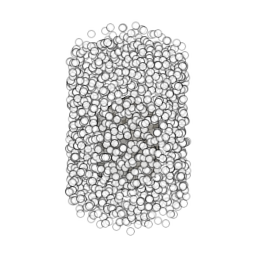
HALS-Total (Autodesk Fusion 360 archive; units mm, degrees)
design "PointCloud-1443points"
Autodesk Fusion 360 part; units mm, degrees
ref_plane "WorkPlane1" through (0, 0, 1223) normal (0, 0, 1) x (1, 0, 0)
sketch "CSV Points - Sketch1" plane through (0, 0, 0) normal (0, 0, 1) x (1, 0, 0)
  point P0 (142.14, 15.69)
  point P1 (141.12, 15.83)
  point P2 (134.47, 12)
  point P3 (116.13, 14.26)
  point P4 (129.36, 12.91)
  point P5 (124.41, 25.54)
  point P6 (141.97, 34.08)
  point P7 (106.73, 16.52)
  point P8 (125.57, 18.99)
  point P9 (134.24, 31.98)
  point P10 (130.24, 26.97)
  point P11 (146.5, 27.15)
  point P12 (98.71, 25.71)
  point P13 (125.11, 21.83)
  point P14 (125.91, 16.58)
  point P15 (113.34, 24.71)
  point P16 (145.3, 33.01)
  point P17 (131.67, 18.74)
  point P18 (136.19, 22.3)
  point P19 (135.78, 34.11)
  point P20 (143.32, 27.86)
  point P21 (129.53, 25.41)
  point P22 (116.49, 28.83)
  point P23 (141.16, 22.86)
  point P24 (141.54, 20.4)
  point P25 (133.86, 50.31)
  point P26 (128.21, 38.95)
  point P27 (129.84, 36.98)
  point P28 (125.52, 49.7)
  point P29 (133.48, 45.44)
  point P30 (125.98, 42.64)
  point P31 (125.43, 49.92)
  point P32 (137.66, 38.7)
  point P33 (116.67, 35.67)
  point P34 (138.63, 51.83)
  point P35 (122.24, 44.25)
  point P36 (141.15, 44.5)
  point P37 (117.73, 31.99)
  point P38 (104.55, 42.88)
  point P39 (131.17, 42.87)
  point P40 (133.94, 47.17)
  point P41 (123.23, 47.3)
  point P42 (141.02, 41.5)
  point P43 (118.06, 34.52)
  point P44 (109.08, 42.31)
  point P45 (128.64, 62.46)
  point P46 (124.24, 55.32)
  point P47 (109.64, 60.03)
  point P48 (123.56, 67.93)
  point P49 (136.01, 60.84)
  point P50 (113.44, 54.84)
  point P51 (132.76, 67.64)
  point P52 (106.86, 45.14)
  point P53 (124.95, 65.32)
  point P54 (117.03, 67.3)
  point P55 (123.06, 57.91)
  point P56 (129.92, 59.75)
  point P57 (121.97, 68.73)
  point P58 (122.62, 65.47)
  point P59 (118.39, 51.23)
  point P60 (117.24, 58.45)
  point P61 (115.65, 57.16)
  point P62 (132.97, 57.82)
  point P63 (99.49, 53.57)
  point P64 (97.67, 54.81)
  point P65 (114.35, 85.86)
  point P66 (120.7, 87.37)
  point P67 (110.26, 74.37)
  point P68 (94.95, 57.5)
  point P69 (101.04, 60.95)
  point P70 (101.85, 68.96)
  point P71 (103.82, 74.87)
  point P72 (119.64, 90.48)
  point P73 (110.83, 71.7)
  point P74 (101.43, 64.12)
  point P75 (111.81, 79.17)
  point P76 (118.39, 81.98)
  point P77 (125.8, 74.1)
  point P78 (94.34, 58.49)
  point P79 (104.36, 68.81)
  point P80 (97.27, 71.97)
  point P81 (86.12, 63.5)
  point P82 (109.11, 72.49)
  point P83 (126.06, 77.55)
  point P84 (96.39, 93.08)
  point P85 (98.57, 86.29)
  point P86 (97.21, 84.8)
  point P87 (81.73, 79.48)
  point P88 (110.02, 86.58)
  point P89 (95.82, 78.71)
  point P90 (96.7, 89.86)
  point P91 (96.15, 87.49)
  point P92 (87.33, 73.28)
  point P93 (98.24, 75.66)
  point P94 (91.69, 90.74)
  point P95 (111.02, 94.82)
  point P96 (93.93, 83.98)
  point P97 (100.83, 95.68)
  point P98 (108.18, 87.29)
  point P99 (107.7, 86.28)
  point P100 (85.45, 81.38)
  point P101 (97.81, 87.15)
  point P102 (103.86, 89.34)
  point P103 (82.82, 96.28)
  point P104 (99.12, 111.25)
  point P105 (102.06, 107.18)
  point P106 (75.65, 94.43)
  point P107 (72.22, 89.5)
  point P108 (82.6, 87.04)
  point P109 (94.65, 105.86)
  point P110 (71.44, 83.64)
  point P111 (95.66, 96.67)
  point P112 (76.88, 99.83)
  point P113 (93.85, 111.84)
  point P114 (86.15, 94.67)
  point P115 (80.33, 86.44)
  point P116 (85.05, 103.55)
  point P117 (82.87, 105.3)
  point P118 (78.78, 81.01)
  point P119 (86.12, 98.72)
  point P120 (80.36, 91.79)
  point P121 (101.42, 105.02)
  point P122 (60.26, 97.95)
  point P123 (80.8, 121.61)
  point P124 (81.89, 111.08)
  point P125 (85.06, 114.95)
  point P126 (64.96, 98.51)
  point P127 (71.67, 115.59)
  point P128 (61.41, 104.26)
  point P129 (66.04, 95.37)
  point P130 (79.74, 112.63)
  point P131 (78.55, 124.25)
  point P132 (73.87, 114.19)
  point P133 (82.64, 109.27)
  point P134 (81.89, 113.55)
  point P135 (78.49, 115.93)
  point P136 (58.88, 97.61)
  point P137 (73.04, 120.61)
  point P138 (77.17, 114.41)
  point P139 (76.81, 106.12)
  point P140 (83.46, 111.16)
  point P141 (72.43, 129.07)
  point P142 (66.85, 124.15)
  point P143 (53.03, 121.97)
  point P144 (46.97, 95.03)
  point P145 (53.99, 108.29)
  point P146 (56.79, 131.24)
  point P147 (66.41, 124.38)
  point P148 (60.87, 108.03)
  point P149 (52.23, 113.56)
  point P150 (60.46, 128.49)
  point P151 (72.28, 125.7)
  point P152 (50.04, 95.71)
  point P153 (57.2, 135.41)
  point P154 (66.74, 130.98)
  point P155 (64.85, 134.15)
  point P156 (51.86, 115.93)
  point P157 (59.26, 107.79)
  point P158 (66.27, 121.05)
  point P159 (60.6, 136.12)
  point P160 (65.08, 134.03)
  point P161 (53.88, 138.92)
  point P162 (37.33, 127.65)
  point P163 (40.09, 136.22)
  point P164 (41.57, 108.3)
  point P165 (45.84, 130.16)
  point P166 (46.6, 142.58)
  point P167 (48.57, 118.43)
  point P168 (30.94, 113.87)
  point P169 (34.88, 110.63)
  point P170 (39.48, 109.07)
  point P171 (52.18, 139.56)
  point P172 (30.41, 99.46)
  point P173 (36.53, 129.96)
  point P174 (51.39, 129.15)
  point P175 (38.15, 112.72)
  point P176 (41.25, 121.17)
  point P177 (41.97, 105.99)
  point P178 (37.26, 130.8)
  point P179 (41.57, 136.82)
  point P180 (41.52, 110.46)
  point P181 (15.4, 106.9)
  point P182 (21.58, 133.26)
  point P183 (34.83, 140.75)
  point P184 (26.95, 137.38)
  point P185 (21.94, 112.89)
  point P186 (30.94, 123.17)
  point P187 (23.43, 143.09)
  point P188 (18.88, 132.66)
  point P189 (28.8, 126.77)
  point P190 (28.12, 128.97)
  point P191 (18.4, 105.41)
  point P192 (33.02, 126.77)
  point P193 (26.97, 145.52)
  point P194 (26.57, 128.28)
  point P195 (32.44, 136.19)
  point P196 (22.28, 147.32)
  point P197 (22.18, 143.29)
  point P198 (32.45, 135.16)
  point P199 (26.94, 131.26)
  point P200 (8.64, 126.71)
  point P201 (2.61, 135.97)
  point P202 (2.18, 124.98)
  point P203 (9.98, 142.65)
  point P204 (12.32, 123.39)
  point P205 (15.11, 123.08)
  point P206 (6.94, 141.83)
  point P207 (4.68, 121.91)
  point P208 (16.97, 128.89)
  point P209 (11.91, 133.47)
  point P210 (9.78, 121.61)
  point P211 (0.98, 140)
  point P212 (3.65, 122.95)
  point P213 (7.94, 137.77)
  point P214 (15.61, 139.13)
  point P215 (15.47, 140.15)
  point P216 (8.36, 136.74)
  point P217 (3.74, 142.95)
  point P218 (-6.64, 118.81)
  point P219 (-10.91, 148.6)
  point P220 (-12.75, 119.32)
  point P221 (-2.6, 123.97)
  point P222 (-3.64, 148.96)
  point P223 (-12.75, 121.33)
  point P224 (-9.82, 130.63)
  point P225 (-7.57, 139.8)
  point P226 (-16.26, 126.96)
  point P227 (-0.24, 136)
  point P228 (-5.76, 131.87)
  point P229 (-12.3, 143.47)
  point P230 (-12.8, 135.4)
  point P231 (-4.31, 129.93)
  point P232 (-1.44, 117.99)
  point P233 (-16.33, 139.04)
  point P234 (-8.67, 137.73)
  point P235 (-8.91, 137.71)
  point P236 (-15.63, 135.1)
  point P237 (-18.03, 120.66)
  point P238 (-22.14, 110.81)
  point P239 (-26.88, 133.32)
  point P240 (-20.89, 141.47)
  point P241 (-35.81, 140.51)
  point P242 (-33.32, 143.17)
  point P243 (-24.52, 144.94)
  point P244 (-24.08, 133.85)
  point P245 (-27.49, 123.99)
  point P246 (-33.68, 126.6)
  point P247 (-18.19, 132.76)
  point P248 (-30.36, 142.81)
  point P249 (-25.06, 132.65)
  point P250 (-22.93, 143.18)
  point P251 (-32.21, 133.16)
  point P252 (-34.11, 138.87)
  point P253 (-21.04, 134.36)
  point P254 (-28.18, 146.31)
  point P255 (-24.34, 116.49)
  point P256 (-32.54, 116.54)
  point P257 (-39.14, 131.29)
  point P258 (-47.6, 142.25)
  point P259 (-53.76, 137.89)
  point P260 (-50.21, 127.47)
  point P261 (-43.24, 130)
  point P262 (-40.81, 136.01)
  point P263 (-38.22, 137.8)
  point P264 (-41.13, 114.86)
  point P265 (-40.75, 110.74)
  point P266 (-42.82, 137.49)
  point P267 (-41.27, 128.54)
  point P268 (-45.7, 113.12)
  point P269 (-46.52, 122.46)
  point P270 (-46.46, 134.18)
  point P271 (-37.49, 130.73)
  point P272 (-41.6, 144.12)
  point P273 (-48.18, 139.94)
  point P274 (-49.94, 130.79)
  point P275 (-51.49, 102.83)
  point P276 (-61.55, 113.37)
  point P277 (-55.47, 126.36)
  point P278 (-56.09, 127.18)
  point P279 (-70.87, 131.07)
  point P280 (-62.9, 125.07)
  point P281 (-64.15, 134.49)
  point P282 (-60.94, 106.84)
  point P283 (-55.34, 132.94)
  point P284 (-57.26, 123.36)
  point P285 (-58.25, 112.85)
  point P286 (-59.9, 113.12)
  point P287 (-48.33, 106.55)
  point P288 (-58.07, 136.13)
  point P289 (-64.68, 116.21)
  point P290 (-58.74, 120.44)
  point P291 (-60.04, 122.03)
  point P292 (-68.36, 123.32)
  point P293 (-53.79, 124.91)
  point P294 (-56.98, 126.78)
  point P295 (-70.28, 112.91)
  point P296 (-79.36, 110.44)
  point P297 (-86.45, 116.41)
  point P298 (-64.71, 108.12)
  point P299 (-74.35, 111.48)
  point P300 (-72.51, 107.9)
  point P301 (-67.59, 113.38)
  point P302 (-87.46, 116.91)
  point P303 (-80.14, 112.35)
  point P304 (-60.41, 96.68)
  point P305 (-77.04, 120.47)
  point P306 (-84.89, 121.23)
  point P307 (-88.47, 116.14)
  point P308 (-70.42, 121)
  point P309 (-78.53, 114.69)
  point P310 (-79.94, 122.17)
  point P311 (-66.88, 109.14)
  point P312 (-82.49, 113.12)
  point P313 (-88, 120.24)
  point P314 (-71.9, 117.79)
  point P315 (-81.19, 93.73)
  point P316 (-90.62, 111.91)
  point P317 (-80.29, 83.72)
  point P318 (-88.76, 92.23)
  point P319 (-81.99, 100.89)
  point P320 (-80.37, 93.11)
  point P321 (-87.16, 96.46)
  point P322 (-78.63, 101)
  point P323 (-80.55, 87.6)
  point P324 (-95.08, 112.11)
  point P325 (-93.9, 113.1)
  point P326 (-98.65, 100.74)
  point P327 (-71.88, 76.54)
  point P328 (-93.17, 117.55)
  point P329 (-84.82, 95.87)
  point P330 (-89.94, 102.02)
  point P331 (-77.36, 96.91)
  point P332 (-94.64, 100.43)
  point P333 (-98.48, 100.91)
  point P334 (-110.9, 99.51)
  point P335 (-113.21, 98.41)
  point P336 (-87.82, 71.11)
  point P337 (-107, 102.25)
  point P338 (-94.39, 90.84)
  point P339 (-107.72, 87.85)
  point P340 (-111.28, 96.05)
  point P341 (-99.42, 89.84)
  point P342 (-108.1, 84.16)
  point P343 (-106, 97.47)
  point P344 (-91.92, 91.92)
  point P345 (-99.91, 84.73)
  point P346 (-112.33, 93.26)
  point P347 (-103.6, 101.45)
  point P348 (-102.06, 95.84)
  point P349 (-86.09, 68.48)
  point P350 (-106.35, 94.09)
  point P351 (-108.77, 95.89)
  point P352 (-96.13, 76.74)
  point P353 (-113.26, 67.79)
  point P354 (-108.15, 72.13)
  point P355 (-102.21, 68.42)
  point P356 (-115.96, 69.13)
  point P357 (-117.71, 88.06)
  point P358 (-105.02, 74.91)
  point P359 (-126.36, 78.96)
  point P360 (-112.05, 71.66)
  point P361 (-116.32, 81.45)
  point P362 (-90.68, 69.08)
  point P363 (-108.9, 63.38)
  point P364 (-104.79, 71.75)
  point P365 (-117.15, 76.66)
  point P366 (-110.84, 67.92)
  point P367 (-117.16, 85.43)
  point P368 (-120.24, 88)
  point P369 (-115.35, 70.14)
  point P370 (-114.51, 75.22)
  point P371 (-118.96, 81.15)
  point P372 (-116.34, 55.74)
  point P373 (-122.5, 61.34)
  point P374 (-116.77, 63.67)
  point P375 (-97.98, 43.01)
  point P376 (-132.67, 58.51)
  point P377 (-103.8, 56.12)
  point P378 (-104.43, 52.75)
  point P379 (-116.43, 55.54)
  point P380 (-107.71, 61.44)
  point P381 (-129.25, 53.8)
  point P382 (-121.54, 56.42)
  point P383 (-110.19, 56.87)
  point P384 (-98.1, 51.94)
  point P385 (-126.59, 57.42)
  point P386 (-125.1, 53.36)
  point P387 (-122.33, 68.09)
  point P388 (-129.32, 63.35)
  point P389 (-121.13, 59.6)
  point P390 (-120.7, 66.9)
  point P391 (-137.04, 40.85)
  point P392 (-109.06, 36.49)
  point P393 (-122.05, 47.59)
  point P394 (-129.42, 50.72)
  point P395 (-119.56, 39.77)
  point P396 (-142.72, 42.82)
  point P397 (-129.13, 35.81)
  point P398 (-116.82, 41.6)
  point P399 (-122.94, 45.23)
  point P400 (-125.07, 38.96)
  point P401 (-132.35, 42.49)
  point P402 (-113.12, 45.7)
  point P403 (-126.2, 47.94)
  point P404 (-137.96, 47.77)
  point P405 (-139.38, 39.97)
  point P406 (-131.56, 38.22)
  point P407 (-112.58, 38.55)
  point P408 (-136.39, 52.08)
  point P409 (-123.4, 49.61)
  point P410 (-142.14, 33.34)
  point P411 (-143.48, 36.31)
  point P412 (-146.37, 21.88)
  point P413 (-132.38, 26.45)
  point P414 (-116.65, 23.52)
  point P415 (-143.44, 21.18)
  point P416 (-137.54, 35.31)
  point P417 (-121.75, 28.33)
  point P418 (-120.29, 20.35)
  point P419 (-124.99, 22.49)
  point P420 (-136.68, 30.3)
  point P421 (-107.27, 28.54)
  point P422 (-147.62, 20.22)
  point P423 (-134.01, 28.48)
  point P424 (-129.7, 24.51)
  point P425 (-103.71, 16.43)
  point P426 (-113.67, 27.71)
  point P427 (-131.1, 32.2)
  point P428 (-118.56, 18.57)
  point P429 (-125.69, 24.2)
  point P430 (-130.26, 13.92)
  point P431 (-118.97, 2.7)
  point P432 (-146.96, 3.59)
  point P433 (-128.29, 13.48)
  point P434 (-144.59, 10.87)
  point P435 (-126.81, 6.87)
  point P436 (-116.08, 14.66)
  point P437 (-115, 0.2)
  point P438 (-122.88, 5.37)
  point P439 (-135.5, 11.62)
  point P440 (-142.37, 13.46)
  point P441 (-146.91, 5.13)
  point P442 (-138.99, 1.7)
  point P443 (-143.02, 16.8)
  point P444 (-107.79, 6.78)
  point P445 (-136.7, 9.08)
  point P446 (-115.25, 13.13)
  point P447 (-115.99, 1.62)
  point P448 (-112.94, 3.55)
  point P449 (-121.42, 11.91)
  point P450 (-138.02, -16.46)
  point P451 (-122.35, -12.64)
  point P452 (-138.68, -9.45)
  point P453 (-147.97, -2.84)
  point P454 (-144.98, -2.53)
  point P455 (-133.67, -9.35)
  point P456 (-145.28, -14.5)
  point P457 (-148.88, -18.28)
  point P458 (-125.85, -6.16)
  point P459 (-123.91, -4.76)
  point P460 (-145.4, -13.23)
  point P461 (-137.56, -11.07)
  point P462 (-132, -0.92)
  point P463 (-114.95, -3.41)
  point P464 (-115.8, -6.88)
  point P465 (-141.12, -15.83)
  point P466 (-141.14, -15.58)
  point P467 (-143.73, -8.79)
  point P468 (-146.95, -3.85)
  point P469 (-144.64, -35.79)
  point P470 (-124.62, -24.45)
  point P471 (-125.65, -24.42)
  point P472 (-128.99, -32.4)
  point P473 (-123.36, -20.2)
  point P474 (-119.79, -17.05)
  point P475 (-119.94, -27.25)
  point P476 (-117.25, -25.56)
  point P477 (-144.75, -19.06)
  point P478 (-110.33, -19.26)
  point P479 (-131.61, -34.28)
  point P480 (-140.65, -25.81)
  point P481 (-128.28, -26.57)
  point P482 (-137.16, -32.68)
  point P483 (-122.61, -18.54)
  point P484 (-132.42, -20.5)
  point P485 (-118.63, -28.48)
  point P486 (-130.28, -26.74)
  point P487 (-117.95, -22.07)
  point P488 (-138.62, -45.84)
  point P489 (-137.88, -48.01)
  point P490 (-106.28, -41.23)
  point P491 (-120.94, -35.36)
  point P492 (-110.32, -32.47)
  point P493 (-126.03, -48.38)
  point P494 (-133.94, -47.17)
  point P495 (-127.37, -41.63)
  point P496 (-98.07, -40.22)
  point P497 (-127.38, -34.61)
  point P498 (-140.12, -44.45)
  point P499 (-138.22, -50.04)
  point P500 (-113.34, -42.38)
  point P501 (-138.66, -42.39)
  point P502 (-134.71, -38.12)
  point P503 (-123.57, -49.18)
  point P504 (-128.82, -43.6)
  point P505 (-140.1, -47.7)
  point P506 (-105.99, -41.97)
  point P507 (-131.76, -37.53)
  point P508 (-98.13, -42.67)
  point P509 (-119.23, -58.93)
  point P510 (-127.98, -63.81)
  point P511 (-132.16, -57.19)
  point P512 (-96.06, -51.51)
  point P513 (-126.33, -71.18)
  point P514 (-119.01, -54.74)
  point P515 (-124.87, -58.76)
  point P516 (-118.75, -62.08)
  point P517 (-129.98, -54.64)
  point P518 (-117.61, -59.93)
  point P519 (-105.34, -50.92)
  point P520 (-106.8, -47.77)
  point P521 (-106.91, -58.77)
  point P522 (-129.82, -71.07)
  point P523 (-135.2, -60.2)
  point P524 (-125.04, -60.72)
  point P525 (-132.88, -67.41)
  point P526 (-127.26, -75.56)
  point P527 (-125.2, -77.03)
  point P528 (-101.62, -67.51)
  point P529 (-114.29, -84.27)
  point P530 (-119.77, -88.63)
  point P531 (-110.2, -72.66)
  point P532 (-124.08, -76.94)
  point P533 (-114.6, -67.5)
  point P534 (-103.59, -71.73)
  point P535 (-104.59, -73.78)
  point P536 (-103.06, -59.5)
  point P537 (-114.11, -72.14)
  point P538 (-123.42, -79.85)
  point P539 (-115, -86.66)
  point P540 (-97.33, -70.19)
  point P541 (-97.71, -66.16)
  point P542 (-127.58, -76.96)
  point P543 (-100.08, -60.61)
  point P544 (-112.75, -76.05)
  point P545 (-102.88, -74.47)
  point P546 (-103.56, -98.62)
  point P547 (-85.07, -68.15)
  point P548 (-113.62, -91.68)
  point P549 (-96.47, -91.55)
  point P550 (-80.51, -71.99)
  point P551 (-93.39, -80.05)
  point P552 (-97.38, -96.37)
  point P553 (-105.37, -81.15)
  point P554 (-86.56, -72.63)
  point P555 (-101.91, -93.05)
  point P556 (-106.22, -98.7)
  point P557 (-102, -83.78)
  point P558 (-116.31, -91.52)
  point P559 (-88.9, -86.45)
  point P560 (-109.27, -95.32)
  point P561 (-86.53, -75.75)
  point P562 (-81.29, -78.5)
  point P563 (-115.36, -91.11)
  point P564 (-106.02, -86.77)
  point P565 (-86.14, -105.24)
  point P566 (-89.25, -113.01)
  point P567 (-88.92, -92.08)
  point P568 (-94.85, -108.35)
  point P569 (-88.09, -100.98)
  point P570 (-103.18, -106.1)
  point P571 (-89.05, -113.16)
  point P572 (-88.86, -108.18)
  point P573 (-89.86, -96.7)
  point P574 (-70.8, -77.54)
  point P575 (-90.63, -108.01)
  point P576 (-75.05, -97.45)
  point P577 (-92.14, -93.11)
  point P578 (-78.74, -91.87)
  point P579 (-94.65, -105.86)
  point P580 (-80.54, -84.87)
  point P581 (-81.01, -100.39)
  point P582 (-80.03, -99.9)
  point P583 (-99.31, -104.28)
  point P584 (-84.44, -116.65)
  point P585 (-78.85, -116.89)
  point P586 (-74.6, -123.17)
  point P587 (-77.48, -128.44)
  point P588 (-61.11, -90.26)
  point P589 (-80.14, -111.12)
  point P590 (-68.01, -90.25)
  point P591 (-78.22, -120.91)
  point P592 (-73.21, -115.8)
  point P593 (-77.82, -110.31)
  point P594 (-71.16, -102.77)
  point P595 (-65.98, -112.01)
  point P596 (-72.19, -116.44)
  point P597 (-74.31, -112.7)
  point P598 (-75.54, -102.09)
  point P599 (-67.06, -90.95)
  point P600 (-69.17, -104.12)
  point P601 (-78.07, -126.91)
  point P602 (-76.07, -128.12)
  point P603 (-50.22, -98.99)
  point P604 (-57.22, -117.84)
  point P605 (-56.13, -126.07)
  point P606 (-64.83, -118.41)
  point P607 (-71.78, -130.57)
  point P608 (-49.41, -110.45)
  point P609 (-62.24, -128.75)
  point P610 (-56.29, -110.48)
  point P611 (-53.48, -127.22)
  point P612 (-61.16, -116.98)
  point P613 (-73, -126.44)
  point P614 (-62.16, -132.1)
  point P615 (-61.01, -132.64)
  point P616 (-70.2, -124.58)
  point P617 (-54.82, -102.23)
  point P618 (-58.38, -134.91)
  point P619 (-64.25, -128.87)
  point P620 (-55.83, -112.96)
  point P621 (-55.82, -128.39)
  point P622 (-40.82, -143.3)
  point P623 (-48.96, -123.66)
  point P624 (-45.44, -133.48)
  point P625 (-34.95, -103.25)
  point P626 (-47.7, -119.86)
  point P627 (-31.04, -109.69)
  point P628 (-40.93, -133.88)
  point P629 (-39.92, -106.78)
  point P630 (-50.04, -138.22)
  point P631 (-43.54, -137.26)
  point P632 (-38.54, -141.86)
  point P633 (-50.47, -123.05)
  point P634 (-40.39, -123.57)
  point P635 (-48.83, -138.65)
  point P636 (-52.32, -136.3)
  point P637 (-41.22, -140.06)
  point P638 (-41.26, -141.09)
  point P639 (-48.1, -124)
  point P640 (-47.03, -135.05)
  point P641 (-45.84, -138.62)
  point P642 (-25.57, -136.63)
  point P643 (-28.96, -141.06)
  point P644 (-29.41, -122.52)
  point P645 (-20.35, -131.43)
  point P646 (-21.68, -143.37)
  point P647 (-29.2, -122.57)
  point P648 (-28.8, -139.05)
  point P649 (-24.55, -133.77)
  point P650 (-32.52, -124.83)
  point P651 (-24.59, -140.87)
  point P652 (-29.82, -136.79)
  point P653 (-27.03, -118.97)
  point P654 (-18.04, -126.72)
  point P655 (-22.3, -136.19)
  point P656 (-28.99, -115.41)
  point P657 (-24.42, -125.65)
  point P658 (-27.34, -139.34)
  point P659 (-35.55, -143.67)
  point P660 (-3.66, -139.95)
  point P661 (-9.04, -147.72)
  point P662 (-14.7, -133.19)
  point P663 (-16.5, -147.08)
  point P664 (-8.66, -145.74)
  point P665 (-3.59, -120.95)
  point P666 (-0.95, -136)
  point P667 (-11.87, -147.52)
  point P668 (-12.05, -132.45)
  point P669 (-15.79, -119.96)
  point P670 (-5.26, -136.9)
  point P671 (-6.64, -135.84)
  point P672 (-15.84, -129.03)
  point P673 (-13.21, -132.34)
  point P674 (-9.63, -137.66)
  point P675 (-2.53, -144.98)
  point P676 (-2.73, -141.97)
  point P677 (-8.43, -123.71)
  point P678 (-14.6, -141.25)
  point P679 (-16.58, -139.02)
  point P680 (14.15, -144.31)
  point P681 (3.96, -125.94)
  point P682 (1.98, -141.99)
  point P683 (14.6, -128.17)
  point P684 (8.95, -134.7)
  point P685 (9.04, -143.72)
  point P686 (13.77, -117.19)
  point P687 (1.69, -137.99)
  point P688 (4.54, -129.92)
  point P689 (13.55, -143.36)
  point P690 (12.04, -140.48)
  point P691 (6.5, -148.86)
  point P692 (0.22, -127)
  point P693 (15.29, -121.04)
  point P694 (6.98, -128.81)
  point P695 (11.25, -149.58)
  point P696 (14.32, -136.25)
  point P697 (3.25, -132.96)
  point P698 (2.84, -124.97)
  point P699 (14.98, -140.2)
  point P700 (27.42, -142.38)
  point P701 (22.43, -143.25)
  point P702 (27.43, -111.68)
  point P703 (28.18, -115.61)
  point P704 (23.15, -146.18)
  point P705 (26.74, -141.5)
  point P706 (28.9, -135.96)
  point P707 (18.32, -133.75)
  point P708 (26.23, -98.57)
  point P709 (30.3, -136.68)
  point P710 (25.85, -143.69)
  point P711 (21.18, -125.22)
  point P712 (33.09, -142.2)
  point P713 (32.83, -127.85)
  point P714 (20.89, -141.47)
  point P715 (20.16, -99.99)
  point P716 (28.8, -144.15)
  point P717 (21.14, -141.43)
  point P718 (34.59, -136.69)
  point P719 (32.65, -139.22)
  point P720 (39.16, -97.42)
  point P721 (48.52, -127.05)
  point P722 (46, -134.34)
  point P723 (41.29, -142.12)
  point P724 (36.38, -126.89)
  point P725 (42.54, -122.84)
  point P726 (45.45, -119.66)
  point P727 (49.07, -121.46)
  point P728 (38.21, -119.02)
  point P729 (39.55, -126.98)
  point P730 (44.54, -121.07)
  point P731 (40.59, -113.99)
  point P732 (37.95, -136.84)
  point P733 (38.79, -129.31)
  point P734 (39.77, -119.56)
  point P735 (43.06, -109.86)
  point P736 (50.49, -129.51)
  point P737 (42.2, -126.13)
  point P738 (36.28, -121.71)
  point P739 (56.72, -102.33)
  point P740 (64.46, -131)
  point P741 (64.23, -131.11)
  point P742 (65.66, -117.96)
  point P743 (52.57, -123.26)
  point P744 (59.49, -131.14)
  point P745 (52.41, -98.98)
  point P746 (67.88, -131.52)
  point P747 (62.73, -135.15)
  point P748 (57.26, -137.56)
  point P749 (72.83, -127.69)
  point P750 (64.15, -134.49)
  point P751 (51.4, -101.75)
  point P752 (68.01, -125.79)
  point P753 (50.85, -115.28)
  point P754 (55.87, -127.28)
  point P755 (69.41, -127.31)
  point P756 (61.34, -122.5)
  point P757 (63.95, -133.47)
  point P758 (67.06, -98.31)
  point P759 (80.16, -122.03)
  point P760 (67.54, -111.08)
  point P761 (84.46, -115.4)
  point P762 (77.77, -106.65)
  point P763 (69.49, -113.4)
  point P764 (82.13, -125.51)
  point P765 (63.28, -92.41)
  point P766 (62.37, -107.17)
  point P767 (89.08, -116.93)
  point P768 (73.99, -105.67)
  point P769 (75.97, -118.79)
  point P770 (79.49, -127.21)
  point P771 (71.43, -100.14)
  point P772 (75.48, -100.89)
  point P773 (72.2, -121.11)
  point P774 (65.64, -98.06)
  point P775 (78.79, -118.14)
  point P776 (69.33, -115.84)
  point P777 (87.97, -110.19)
  point P778 (87.95, -99.76)
  point P779 (96.74, -109.35)
  point P780 (90.26, -113.48)
  point P781 (85.57, -91.12)
  point P782 (87.46, -89.31)
  point P783 (91.98, -110.79)
  point P784 (92.49, -109.06)
  point P785 (92.73, -100.85)
  point P786 (78.01, -100.21)
  point P787 (93.19, -103.13)
  point P788 (95.4, -110.52)
  point P789 (91.64, -112.37)
  point P790 (89.45, -92.95)
  point P791 (100.18, -104.83)
  point P792 (94.4, -116.57)
  point P793 (66.92, -76.98)
  point P794 (98.17, -109.41)
  point P795 (103.78, -101.27)
  point P796 (96.79, -91.21)
  point P797 (91.44, -72.99)
  point P798 (94.51, -83.33)
  point P799 (109.35, -96.74)
  point P800 (108.15, -85.72)
  point P801 (102.78, -96.52)
  point P802 (75.02, -73.46)
  point P803 (106.18, -88.15)
  point P804 (99.15, -84.08)
  point P805 (98.99, -98.99)
  point P806 (97.9, -90.02)
  point P807 (112.05, -87.23)
  point P808 (109.07, -98.55)
  point P809 (77.21, -66.65)
  point P810 (97.01, -78.83)
  point P811 (76.38, -73.5)
  point P812 (77.95, -74.75)
  point P813 (108.8, -88.1)
  point P814 (99.02, -85.77)
  point P815 (97.3, -59.4)
  point P816 (109.75, -80.32)
  point P817 (102.61, -74.83)
  point P818 (109.14, -66.88)
  point P819 (103.76, -67.9)
  point P820 (103.14, -70.62)
  point P821 (108.03, -62.88)
  point P822 (106.59, -81.2)
  point P823 (120.42, -84.32)
  point P824 (115.42, -73.81)
  point P825 (123.82, -77.37)
  point P826 (121.3, -86.52)
  point P827 (95.29, -71.28)
  point P828 (116.82, -69.64)
  point P829 (94.62, -63.58)
  point P830 (118.97, -79.34)
  point P831 (119.27, -71.38)
  point P832 (112.39, -83.47)
  point P833 (120.19, -86.36)
  point P834 (120.55, -75.04)
  point P835 (135.91, -61.08)
  point P836 (119.4, -51.42)
  point P837 (108.45, -60.12)
  point P838 (115.75, -56.95)
  point P839 (113.25, -55.23)
  point P840 (120.58, -67.11)
  point P841 (124.18, -52.97)
  point P842 (119.3, -54.12)
  point P843 (121.08, -64.11)
  point P844 (116.41, -60.08)
  point P845 (118.82, -55.16)
  point P846 (129.25, -53.8)
  point P847 (127.69, -72.83)
  point P848 (110.12, -52.52)
  point P849 (116.14, -58.41)
  point P850 (111.72, -60.4)
  point P851 (134.5, -59.32)
  point P852 (106.22, -46.63)
  point P853 (114.25, -62.03)
  point P854 (94.78, -47.46)
  point P855 (131.72, -50.3)
  point P856 (128.59, -44.28)
  point P857 (143.16, -41.32)
  point P858 (131.69, -37.76)
  point P859 (108.67, -37.63)
  point P860 (100.03, -38)
  point P861 (117.75, -47.58)
  point P862 (114.26, -36.68)
  point P863 (117.44, -36.58)
  point P864 (102.3, -37.64)
  point P865 (133.69, -47.87)
  point P866 (104.07, -28.86)
  point P867 (136.01, -40.81)
  point P868 (141.38, -47.03)
  point P869 (110.72, -43.61)
  point P870 (132.3, -51.58)
  point P871 (110.01, -36.81)
  point P872 (143.75, -42.85)
  point P873 (134.84, -37.65)
  point P874 (136.06, -28.42)
  point P875 (137.47, -26.47)
  point P876 (131.4, -20.58)
  point P877 (145.67, -35.78)
  point P878 (131.21, -31.74)
  point P879 (130.34, -20.88)
  point P880 (128.72, -24.32)
  point P881 (131.07, -27.86)
  point P882 (128.8, -17.64)
  point P883 (120.8, -32.14)
  point P884 (143.52, -31.82)
  point P885 (116.14, -20.9)
  point P886 (137.05, -23.18)
  point P887 (135.38, -31.5)
  point P888 (139.54, -35.57)
  point P889 (148.39, -21.91)
  point P890 (131.36, -26.49)
  point P891 (139.25, -27.82)
  point P892 (145.39, -21.73)
  point P893 (116.22, -13.45)
  point P894 (106.27, -12.48)
  point P895 (148.34, -14.02)
  point P896 (122, -15.63)
  point P897 (139.23, -14.63)
  point P898 (144.18, -15.41)
  point P899 (139.33, -13.66)
  point P900 (84.35, -10.51)
  point P901 (18.93, -1.66)
  point P902 (56.58, -12.75)
  point P903 (63.81, -16.86)
  point P904 (89.15, -12.37)
  point P905 (132.16, -22.12)
  point P906 (137.74, -25.03)
  point P907 (146.04, -34.25)
  point P908 (145.42, -36.8)
  point P909 (124.59, -40.48)
  point P910 (115.05, -46.25)
  point P911 (109.86, -34.01)
  point P912 (89.55, -31.71)
  point P913 (74.09, -27.41)
  point P914 (34.21, -14.1)
  point P915 (34.41, -16.12)
  point P916 (69.37, -35.65)
  point P917 (84.76, -45.07)
  point P918 (112.28, -63.52)
  point P919 (132.57, -63.52)
  point P920 (125.37, -82.35)
  point P921 (109.04, -74.39)
  point P922 (112.13, -65.78)
  point P923 (101.96, -77.39)
  point P924 (56.38, -36.2)
  point P925 (45.98, -31.96)
  point P926 (11.06, -10.13)
  point P927 (65.49, -55.74)
  point P928 (68.58, -56.73)
  point P929 (100.08, -78.19)
  point P930 (111.65, -100.17)
  point P931 (97.78, -100.2)
  point P932 (92.59, -98.25)
  point P933 (86.85, -102.05)
  point P934 (77.13, -93.23)
  point P935 (60.95, -78.01)
  point P936 (48.24, -52.09)
  point P937 (36, -36.13)
  point P938 (15.04, -23.61)
  point P939 (25.88, -36.82)
  point P940 (45.34, -59.74)
  point P941 (42, -71.59)
  point P942 (66.58, -106.97)
  point P943 (82.28, -114.5)
  point P944 (89.64, -120.27)
  point P945 (58.68, -110.37)
  point P946 (50.2, -111.19)
  point P947 (52.11, -101.39)
  point P948 (44.7, -103.78)
  point P949 (45.3, -80.07)
  point P950 (23.93, -57.2)
  point P951 (25.59, -55.37)
  point P952 (7.76, -28.98)
  point P953 (24.11, -78.38)
  point P954 (28.74, -88.45)
  point P955 (34.42, -123.28)
  point P956 (44.4, -125.37)
  point P957 (51.69, -139.75)
  point P958 (29.28, -138.95)
  point P959 (16.36, -117.87)
  point P960 (16.17, -96.66)
  point P961 (13.59, -74.78)
  point P962 (9.45, -42.97)
  point P963 (0, -8)
  point P964 (2.36, -51.95)
  point P965 (5.74, -69.76)
  point P966 (6.98, -124.81)
  point P967 (9.52, -129.65)
  point P968 (18.29, -146.87)
  point P969 (-1.14, -131)
  point P970 (-9.34, -118.63)
  point P971 (-4.45, -87.89)
  point P972 (-3.19, -86.94)
  point P973 (-7.37, -54.5)
  point P974 (-11.57, -67.01)
  point P975 (-24.29, -93.91)
  point P976 (-26.83, -125.16)
  point P977 (-19.54, -135.6)
  point P978 (-22.06, -136.22)
  point P979 (-31.48, -137.44)
  point P980 (-52.78, -140.41)
  point P981 (-35.47, -116.73)
  point P982 (-30.23, -74.07)
  point P983 (-20.32, -74.27)
  point P984 (-11.96, -38.17)
  point P985 (-12.03, -32.87)
  point P986 (-29.32, -51.2)
  point P987 (-29.75, -56.67)
  point P988 (-37.12, -87.45)
  point P989 (-59.74, -110.94)
  point P990 (-53.5, -117.39)
  point P991 (-60.26, -127.48)
  point P992 (-73.41, -130.81)
  point P993 (-77.34, -119.09)
  point P994 (-73.54, -116.77)
  point P995 (-78.05, -103.96)
  point P996 (-51.54, -75)
  point P997 (-48.66, -68.47)
  point P998 (-13.39, -17.45)
  point P999 (-30.92, -36.72)
  point P1000 (-49.04, -54.08)
  point P1001 (-84.96, -86.16)
  point P1002 (-84.77, -98.56)
  point P1003 (-92.47, -103.78)
  point P1004 (-102.53, -101.11)
  point P1005 (-106.9, -91.95)
  point P1006 (-103.78, -92.47)
  point P1007 (-54.08, -49.04)
  point P1008 (-36.72, -30.92)
  point P1009 (-17.45, -13.39)
  point P1010 (-68.47, -48.66)
  point P1011 (-75, -51.54)
  point P1012 (-103.16, -66.99)
  point P1013 (-115.93, -73)
  point P1014 (-118.35, -88.86)
  point P1015 (-125.91, -67.79)
  point P1016 (-124.76, -58.98)
  point P1017 (-119.47, -67.05)
  point P1018 (-114.66, -52.25)
  point P1019 (-87.45, -37.12)
  point P1020 (-56.67, -29.75)
  point P1021 (-51.2, -29.32)
  point P1022 (-32.87, -12.03)
  point P1023 (-38.17, -11.96)
  point P1024 (-74.27, -20.32)
  point P1025 (-74.07, -30.23)
  point P1026 (-137.6, -51.72)
  point P1027 (-141.61, -43.02)
  point P1028 (-146.1, -23.66)
  point P1029 (-143.73, -30.81)
  point P1030 (-140.55, -20.25)
  point P1031 (-119.9, -27.46)
  point P1032 (-93.91, -24.29)
  point P1033 (-67.01, -11.57)
  point P1034 (-54.5, -7.37)
  point P1035 (-8, 0)
  point P1036 (-86.94, -3.19)
  point P1037 (-87.89, -4.45)
  point P1038 (-120, -1.05)
  point P1039 (-136.58, -10.75)
  point P1040 (-148.85, 18.54)
  point P1041 (-138.78, 7.76)
  point P1042 (-128.65, 9.45)
  point P1043 (-69.76, 5.74)
  point P1044 (-51.95, 2.36)
  point P1045 (-28.98, 7.76)
  point P1046 (-42.97, 9.45)
  point P1047 (-74.78, 13.59)
  point P1048 (-96.66, 16.17)
  point P1049 (-104, 14.43)
  point P1050 (-125.25, 26.39)
  point P1051 (-128.49, 47.53)
  point P1052 (-115.58, 32.27)
  point P1053 (-110.29, 39.06)
  point P1054 (-88.45, 28.74)
  point P1055 (-78.38, 24.11)
  point P1056 (-55.37, 25.59)
  point P1057 (-57.2, 23.93)
  point P1058 (-80.07, 45.3)
  point P1059 (-115.75, 52.26)
  point P1060 (-114.78, 61.03)
  point P1061 (-127.66, 54.98)
  point P1062 (-128.97, 66.28)
  point P1063 (-103.43, 77.09)
  point P1064 (-101.03, 62.88)
  point P1065 (-87.71, 63.02)
  point P1066 (-71.59, 42)
  point P1067 (-59.74, 45.34)
  point P1068 (-36.82, 25.88)
  point P1069 (-23.61, 15.04)
  point P1070 (-36.13, 36)
  point P1071 (-52.09, 48.24)
  point P1072 (-78.01, 60.95)
  point P1073 (-81.51, 76.81)
  point P1074 (-100.91, 98.48)
  point P1075 (-111.18, 94.63)
  point P1076 (-115.58, 95.61)
  point P1077 (-88.04, 112.69)
  point P1078 (-94.83, 105.69)
  point P1079 (-56.73, 68.58)
  point P1080 (-55.74, 65.49)
  point P1081 (-10.13, 11.06)
  point P1082 (-31.96, 45.98)
  point P1083 (-36.2, 56.38)
  point P1084 (-70.34, 119.89)
  point P1085 (-86.46, 113.9)
  point P1086 (-78.51, 119.52)
  point P1087 (-82.84, 121.44)
  point P1088 (-72.88, 128.81)
  point P1089 (-54.87, 114.53)
  point P1090 (-45.07, 84.76)
  point P1091 (-35.65, 69.37)
  point P1092 (-16.12, 34.41)
  point P1093 (-14.1, 34.21)
  point P1094 (-27.41, 74.09)
  point P1095 (-31.71, 89.55)
  point P1096 (-45.5, 113.2)
  point P1097 (-37.26, 120.37)
  point P1098 (-44.19, 136)
  point P1099 (-24.26, 144.98)
  point P1100 (-30.83, 131.43)
  point P1101 (-23.78, 130.86)
  point P1102 (-31.64, 125.06)
  point P1103 (-12.37, 89.15)
  point P1104 (-16.86, 63.81)
  point P1105 (-12.75, 56.58)
  point P1106 (-1.66, 18.93)
  point P1107 (-2.09, 49.96)
  point P1108 (-0.38, 72)
  point P1109 (-10.51, 84.35)
  point P1110 (-11.22, 114.45)
  point P1111 (-4.33, 137.93)
  point P1112 (-2.02, 144.99)
  point P1113 (16.46, 138.02)
  point P1114 (6.83, 134.83)
  point P1115 (4.87, 132.91)
  point P1116 (13.24, 130.33)
  point P1117 (7.85, 99.69)
  point P1118 (6.84, 73.68)
  point P1119 (6.05, 46.61)
  point P1120 (4.34, 24.62)
  point P1121 (17.4, 81.16)
  point P1122 (20.7, 89.64)
  point P1123 (20.79, 111.07)
  point P1124 (34.05, 131.67)
  point P1125 (48.67, 139.77)
  point P1126 (55.54, 136.1)
  point P1127 (44.98, 136.8)
  point P1128 (37.21, 136)
  point P1129 (21.34, 59.28)
  point P1130 (18.24, 57.16)
  point P1131 (15.19, 29.3)
  point P1132 (34.74, 73.17)
  point P1133 (38.98, 85.54)
  point P1134 (46.11, 108.62)
  point P1135 (54.29, 107.02)
  point P1136 (84, 118.19)
  point P1137 (70.76, 119.64)
  point P1138 (74.39, 107.83)
  point P1139 (53.37, 82.19)
  point P1140 (40.5, 64.31)
  point P1141 (21.06, 36.34)
  point P1142 (34.57, 41.49)
  point P1143 (42.29, 54.52)
  point P1144 (61.79, 62.66)
  point P1145 (80.44, 98.28)
  point P1146 (79.33, 100.45)
  point P1147 (92.07, 98.73)
  point P1148 (103.12, 96.16)
  point P1149 (105.94, 83.67)
  point P1150 (81.25, 66.5)
  point P1151 (62.66, 61.79)
  point P1152 (54.52, 42.29)
  point P1153 (41.49, 34.57)
  point P1154 (36.34, 21.06)
  point P1155 (64.31, 40.5)
  point P1156 (82.19, 53.37)
  point P1157 (105.36, 72.68)
  point P1158 (118.78, 70.25)
  point P1159 (113.3, 80.52)
  point P1160 (119.5, 60.63)
  point P1161 (109.54, 46.5)
  point P1162 (85.54, 38.98)
  point P1163 (73.17, 34.74)
  point P1164 (29.3, 15.19)
  point P1165 (57.16, 18.24)
  point P1166 (59.28, 21.34)
  point P1167 (127.3, 41.85)
  point P1168 (125.92, 51.39)
  point P1169 (133.16, 46.37)
  point P1170 (136.97, 37.47)
  point P1171 (125.86, 32.55)
  point P1172 (116.97, 21.89)
  point P1173 (89.64, 20.7)
  point P1174 (81.16, 17.4)
  point P1175 (24.62, 4.34)
  point P1176 (46.61, 6.05)
  point P1177 (73.68, 6.84)
  point P1178 (116.18, 13.85)
  point P1179 (134.31, 13.64)
  point P1180 (143.79, 18.68)
  point P1181 (135.42, 12.56)
  point P1182 (73.68, 6.84)
  point P1183 (46.61, 6.05)
  point P1184 (81.16, 17.4)
  point P1185 (89.64, 20.7)
  point P1186 (116.36, 24.94)
  point P1187 (129.01, 22.75)
  point P1188 (141.28, 32.62)
  point P1189 (134.33, 42.87)
  point P1190 (103.5, 37.26)
  point P1191 (59.28, 21.34)
  point P1192 (57.16, 18.24)
  point P1193 (73.17, 34.74)
  point P1194 (85.54, 38.98)
  point P1195 (112.75, 58.45)
  point P1196 (114.72, 54.47)
  point P1197 (124.66, 56.81)
  point P1198 (125.45, 72.72)
  point P1199 (120.77, 78.43)
  point P1200 (115.93, 73)
  point P1201 (82.19, 53.37)
  point P1202 (64.31, 40.5)
  point P1203 (36.34, 21.06)
  point P1204 (41.49, 34.57)
  point P1205 (54.52, 42.29)
  point P1206 (62.66, 61.79)
  point P1207 (91.85, 90.58)
  point P1208 (104.3, 80.9)
  point P1209 (112.94, 94.1)
  point P1210 (92.18, 110.63)
  point P1211 (97.6, 98.97)
  point P1212 (67.42, 86.92)
  point P1213 (61.79, 62.66)
  point P1214 (42.29, 54.52)
  point P1215 (34.57, 41.49)
  point P1216 (21.06, 36.34)
  point P1217 (40.5, 64.31)
  point P1218 (53.37, 82.19)
  point P1219 (60.22, 95.62)
  point P1220 (74.07, 114.06)
  point P1221 (71.72, 123.72)
  point P1222 (60.13, 131.94)
  point P1223 (57.05, 120.14)
  point P1224 (55.22, 106.54)
  point P1225 (38.98, 85.54)
  point P1226 (34.74, 73.17)
  point P1227 (18.24, 57.16)
  point P1228 (21.34, 59.28)
  point P1229 (49.46, 137.37)
  point P1230 (45.6, 142.9)
  point P1231 (33.52, 145.18)
  point P1232 (22.23, 126.06)
  point P1233 (24.53, 114.4)
  point P1234 (20.7, 89.64)
  point P1235 (17.4, 81.16)
  point P1236 (6.05, 46.61)
  point P1237 (6.84, 73.68)
  point P1238 (7.85, 99.69)
  point P1239 (17.13, 131.89)
  point P1240 (1.46, 138.99)
  point P1241 (12.84, 138.41)
  point P1242 (10.98, 139.57)
  point P1243 (-0.79, 150)
  point P1244 (-5.86, 139.88)
  point P1245 (-16.32, 130.99)
  point P1246 (-9.76, 111.57)
  point P1247 (-10.51, 84.35)
  point P1248 (-0.38, 72)
  point P1249 (-2.09, 49.96)
  point P1250 (-12.75, 56.58)
  point P1251 (-16.86, 63.81)
  point P1252 (-12.37, 89.15)
  point P1253 (-31.93, 120.85)
  point P1254 (-30.34, 134.62)
  point P1255 (-19.79, 142.63)
  point P1256 (-52.59, 127.59)
  point P1257 (-44.4, 125.37)
  point P1258 (-44.41, 120.05)
  point P1259 (-31.71, 89.55)
  point P1260 (-27.41, 74.09)
  point P1261 (-14.1, 34.21)
  point P1262 (-16.12, 34.41)
  point P1263 (-35.65, 69.37)
  point P1264 (-45.07, 84.76)
  point P1265 (-45.81, 97.8)
  point P1266 (-53.52, 100.66)
  point P1267 (-63.54, 123.63)
  point P1268 (-77.25, 120.34)
  point P1269 (-75.33, 108.39)
  point P1270 (-36.2, 56.38)
  point P1271 (-31.96, 45.98)
  point P1272 (-55.74, 65.49)
  point P1273 (-56.73, 68.58)
  point P1274 (-79.07, 92.91)
  point P1275 (-95.26, 103.96)
  point P1276 (-93.7, 113.27)
  point P1277 (-99.17, 98.82)
  point P1278 (-103.23, 80.65)
  point P1279 (-90.25, 83.57)
  point P1280 (-78.01, 60.95)
  point P1281 (-52.09, 48.24)
  point P1282 (-36.13, 36)
  point P1283 (-36.82, 25.88)
  point P1284 (-59.74, 45.34)
  point P1285 (-71.59, 42)
  point P1286 (-98.77, 74.97)
  point P1287 (-112.99, 66.29)
  point P1288 (-113.01, 72)
  point P1289 (-120.27, 84.53)
  point P1290 (-123.46, 57.05)
  point P1291 (-120.85, 50.55)
  point P1292 (-105.31, 59.58)
  point P1293 (-80.07, 45.3)
  point P1294 (-57.2, 23.93)
  point P1295 (-55.37, 25.59)
  point P1296 (-78.38, 24.11)
  point P1297 (-88.45, 28.74)
  point P1298 (-129.99, 39.99)
  point P1299 (-142.66, 46.35)
  point P1300 (-145.61, 26.46)
  point P1301 (-137.09, 22.94)
  point P1302 (-127.5, 34.16)
  point P1303 (-100.6, 22.12)
  point P1304 (-96.66, 16.17)
  point P1305 (-74.78, 13.59)
  point P1306 (-42.97, 9.45)
  point P1307 (-51.95, 2.36)
  point P1308 (-69.76, 5.74)
  point P1309 (-119.88, 5.44)
  point P1310 (-121.59, 10)
  point P1311 (-117.85, -5.97)
  point P1312 (-112.92, -4.14)
  point P1313 (-100, 0)
  point P1314 (-87.89, -4.45)
  point P1315 (-86.94, -3.19)
  point P1316 (-54.5, -7.37)
  point P1317 (-67.01, -11.57)
  point P1318 (-93.91, -24.29)
  point P1319 (-125.86, -32.55)
  point P1320 (-135.76, -18.36)
  point P1321 (-136.97, -23.66)
  point P1322 (-138.88, -56.68)
  point P1323 (-132.41, -48.46)
  point P1324 (-133.59, -41.87)
  point P1325 (-132.14, -36.15)
  point P1326 (-74.07, -30.23)
  point P1327 (-74.27, -20.32)
  point P1328 (-38.17, -11.96)
  point P1329 (-51.2, -29.32)
  point P1330 (-56.67, -29.75)
  point P1331 (-87.45, -37.12)
  point P1332 (-97.57, -41.42)
  point P1333 (-122.18, -64.15)
  point P1334 (-122.35, -70.07)
  point P1335 (-108.78, -74.77)
  point P1336 (-103.52, -73.57)
  point P1337 (-75, -51.54)
  point P1338 (-68.47, -48.66)
  point P1339 (-36.72, -30.92)
  point P1340 (-54.08, -49.04)
  point P1341 (-100.01, -90.68)
  point P1342 (-98.57, -92.24)
  point P1343 (-115.83, -88.88)
  point P1344 (-113.21, -95.33)
  point P1345 (-99.41, -109.64)
  point P1346 (-95.66, -102.22)
  point P1347 (-88.89, -105.56)
  point P1348 (-49.04, -54.08)
  point P1349 (-30.92, -36.72)
  point P1350 (-48.66, -68.47)
  point P1351 (-51.54, -75)
  point P1352 (-83.4, -108.69)
  point P1353 (-80.43, -117.03)
  point P1354 (-86.89, -122.27)
  point P1355 (-72.56, -126.69)
  point P1356 (-50.01, -117.82)
  point P1357 (-55.78, -106.25)
  point P1358 (-37.12, -87.45)
  point P1359 (-29.75, -56.67)
  point P1360 (-29.32, -51.2)
  point P1361 (-11.96, -38.17)
  point P1362 (-20.32, -74.27)
  point P1363 (-30.23, -74.07)
  point P1364 (-36.18, -115.46)
  point P1365 (-35.1, -128.29)
  point P1366 (-46.05, -125.84)
  point P1367 (-54.79, -134.25)
  point P1368 (-20.1, -148.65)
  point P1369 (-34.8, -134.57)
  point P1370 (-21.62, -125.15)
  point P1371 (-24.29, -93.91)
  point P1372 (-11.57, -67.01)
  point P1373 (-7.37, -54.5)
  point P1374 (-3.19, -86.94)
  point P1375 (-4.45, -87.89)
  point P1376 (-6.43, -126.84)
  point P1377 (-4.87, -132.91)
  point P1378 (11.31, -137.54)
  point P1379 (0, -131)
  point P1380 (5.81, -127.87)
  point P1381 (5.74, -69.76)
  point P1382 (2.36, -51.95)
  point P1383 (9.45, -42.97)
  point P1384 (13.59, -74.78)
  point P1385 (16.17, -96.66)
  point P1386 (18.32, -109.48)
  point P1387 (24.69, -112.32)
  point P1388 (23.6, -129.87)
  point P1389 (36.23, -135.23)
  point P1390 (35.23, -108.42)
  point P1391 (32.34, -105.14)
  point P1392 (28.74, -88.45)
  point P1393 (24.11, -78.38)
  point P1394 (25.59, -55.37)
  point P1395 (23.93, -57.2)
  point P1396 (45.3, -80.07)
  point P1397 (57.46, -124.37)
  point P1398 (67.95, -120.11)
  point P1399 (57.89, -138.38)
  point P1400 (88.88, -117.09)
  point P1401 (72.54, -113.86)
  point P1402 (69.58, -99)
  point P1403 (60.22, -102.64)
  point P1404 (42, -71.59)
  point P1405 (45.34, -59.74)
  point P1406 (25.88, -36.82)
  point P1407 (36, -36.13)
  point P1408 (48.24, -52.09)
  point P1409 (60.95, -78.01)
  point P1410 (88.23, -88.54)
  point P1411 (93.76, -101.25)
  point P1412 (86.81, -111.11)
  point P1413 (112.71, -95.92)
  point P1414 (109.12, -99.99)
  point P1415 (104.79, -86.69)
  point P1416 (68.58, -56.73)
  point P1417 (65.49, -55.74)
  point P1418 (45.98, -31.96)
  point P1419 (56.38, -36.2)
  point P1420 (111.92, -71.85)
  point P1421 (115.78, -80.47)
  point P1422 (128.08, -65.82)
  point P1423 (120.96, -64.32)
  point P1424 (113.2, -53.02)
  point P1425 (84.76, -45.07)
  point P1426 (69.37, -35.65)
  point P1427 (34.41, -16.12)
  point P1428 (34.21, -14.1)
  point P1429 (74.09, -27.41)
  point P1430 (89.55, -31.71)
  point P1431 (108.4, -38.39)
  point P1432 (123.89, -51.06)
  point P1433 (126.62, -46.84)
  point P1434 (145.02, -38.32)
  point P1435 (144.61, -20.07)
  point P1436 (111.21, -25.06)
  point P1437 (89.15, -12.37)
  point P1438 (63.81, -16.86)
  point P1439 (56.58, -12.75)
  point P1440 (84.35, -10.51)
  point P1441 (116.1, -14.46)
  point P1442 (147.44, -12.9)
box "BoxPrimitive1" add length 110 width 110 height 190 placed x (0, 1, 0) y (-1, 0, 0) z (0, 0, 1) at (110, 0, 0) makes body 1
move_body "Move1" bodies 1 to x (1, 0, 0) y (0, 1, 0) z (0, 0, 1) at (-55, -55, 0)
move_body "Move2" bodies 1 to x (1, 0, 0) y (0, 1, 0) z (0, 0, 1) at (0, 0, 1078)
cylinder "CylinderPrimitive1" add diameter 12 height 1 placed x (0, 0, -1) y (0, 1, 0) z (1, 0, 0) at (55, 0, 1078) separate body makes body 2
move_body "Move3" bodies 2 to x (1, 0, 0) y (0, 1, 0) z (0, 0, 1) at (0, 0, 144)
cylinder "CylinderPrimitive2" add diameter 82 height 10 placed x (0, 0, -1) y (0, 1, 0) z (1, 0, 0) at (55, 0, 1078) separate body makes body 3
move_body "Move4" bodies 3 to x (1, 0, 0) y (0, 1, 0) z (0, 0, 1) at (0, 0, 80)
move_body "Move5" bodies 2 3 to x (1, 0, 0) y (0, 1, 0) z (0, 0, 1) at (-5, 0, 0)
move_body "Move6" bodies 2 to x (1, 0, 0) y (0, 1, 0) z (0, 0, 1) at (2, 0, 0)
move_body "Move7" bodies 2 to x (1, 0, 0) y (0, 1, 0) z (0, 0, 1) at (5, 0, 0)
move_body "Move8" bodies 2 to x (1, 0, 0) y (0, 1, 0) z (0, 0, 1) at (1, 0, 0)

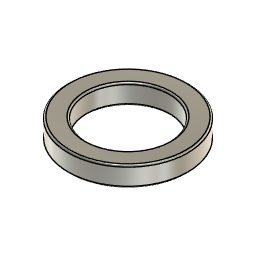
design "Kogellager 72x50x12 6910-2RS"
Autodesk Fusion 360 part; units mm, degrees
cylinder "CylinderPrimitive1" add diameter 72 height 12 placed x (1, 0, 0) y (0, 1, 0) z (0, 0, 1) at (0, 0, 0)
hole "Hole1" at (0, 0, 12) direction (0, 0, -1) diameter 50 depth 12 tip angle 180
fillet "Fillet1" radius 1 4 edges at (-33.5638, -13.0182, 12) (-23.3082, 9.0404, 12) (-33.5638, 13.0182, 0) (-23.3082, -9.0404, 0)
